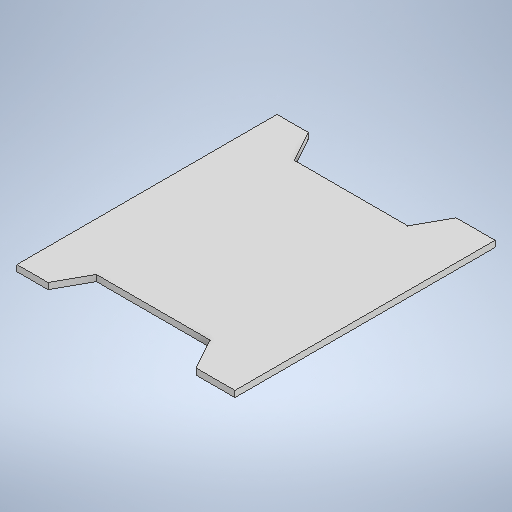
# Autodesk Inventor part: plytka
Saved by Autodesk Inventor 2025 (Build 290162000, 162)
## iProperties
Created: 2025-03-18
Part Number: plytka
Material: Generic
Document SubType Name: Modeling
Designer: HP
Density: 1 g/cm^3
Appearance: Default
Author: HP
Autodesk Inventor part; units mm, degrees
ref_plane "YZ Plane" through (0, 0, 0) normal (1, 0, 0) x (0, 1, 0)
ref_plane "XZ Plane" through (0, 0, 0) normal (0, 1, 0) x (-1, 0, 0)
ref_plane "XY Plane" through (0, 0, 0) normal (0, 0, 1) x (1, 0, 0)
sketch "Sketch1" plane through (0, 0, 0) normal (0, 1, 0) x (-1, 0, 0)
  line L0 (0, -41.75) -> (0, -83.5)
  line L1 (0, -83.5) -> (12.5, -83.5)
  line L2 (18, -73.5) -> (54.5, -73.5)
  line L3 (70, -83.5) -> (70, -41.75)
  line L4 (70, -83.5) -> (60, -83.5)
  line L5 (60, -83.5) -> (54.5, -73.5)
  line L6 (18, -73.5) -> (12.5, -83.5)
  line L7 (0, -41.75) -> (0, 0)
  line L8 (0, 0) -> (12.5, 0)
  line L9 (18, -10) -> (54.5, -10)
  line L10 (70, 0) -> (70, -41.75)
  line L11 (70, 0) -> (60, 0)
  line L12 (60, 0) -> (54.5, -10)
  line L13 (18, -10) -> (12.5, 0)
  constraints: 28 end point, 2 point on line, 1 perpendicular, 1 vertical
extrude "Extrusion1" add sketch "Sketch1" along normal blind 2
body "Solid1"
